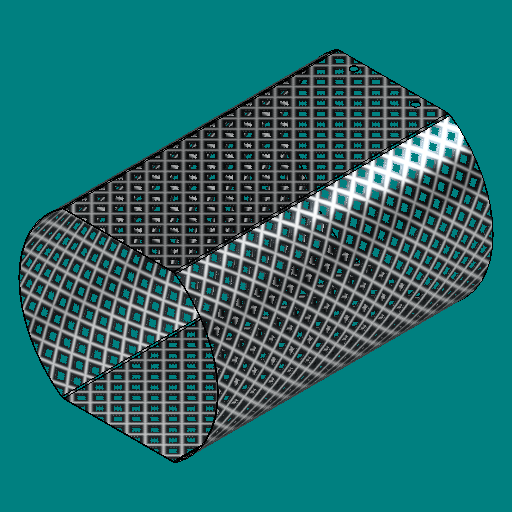
# Autodesk Inventor part: probe-side-large-mesh
Saved by Autodesk Inventor 2025 (Build 290162000, 162)
## iProperties
Created: 2024-05-22
Part Number: probe-side-large-mesh
Material: Stainless Steel
Document SubType Name: Modeling
Designer: kuzmin
Density: 8 g/cm^3
Appearance: Expanded Metal 02
Author: kuzmin
Autodesk Inventor part; units mm, degrees
ref_plane "YZ Plane" through (0, 0, 0) normal (1, 0, 0) x (0, 1, 0)
ref_plane "XZ Plane" through (0, 0, 0) normal (0, 1, 0) x (-1, 0, 0)
ref_plane "XY Plane" through (0, 0, 0) normal (0, 0, 1) x (1, 0, 0)
sketch "Sketch1" plane through (0, 0, 0) normal (0, 0, 1) x (1, 0, 0)
  circle A0 centre (0, 0) radius 28.8
  line L0 (-50, 23.8) -> (50, 23.8)
  line L1 (50, 23.8) -> (50, -23.8)
  line L2 (50, -23.8) -> (-50, -23.8)
  line L3 (-50, -23.8) -> (-50, 23.8)
  point P0 (50, 0)
  point P1 (0, 23.8)
  point P2 (-16.217275, -23.8)
  point P3 (16.217275, -23.8)
  point P4 (16.217275, 23.8)
  point P5 (-16.217275, 23.8)
  dimension "d0" = 57.6
  dimension "d1" = 47.6
  dimension "d2" = 100
  constraints: 8 end point, 2 midpoint, 2 parallel, 1 centre point, 1 coincident, 1 horizontal, 1 horizontal alignment, 1 perpendicular, 1 vertical alignment
  measures "d0" diameter of A0
  measures "d1" distance between parallel lines of L2 L0
  measures "d2" distance of L0.start L0.end
sketch "Sketch1 outline for Extrusion1" plane through (0, 0, 0) normal (0, 0, 1) x (1, 0, 0)
  line L0 (-16.217275, -23.8) -> (16.217275, -23.8)
  arc A0 (-16.217275, 23.8) -> (-16.217275, -23.8) centre (0, 0) ccw
  line L1 (16.217275, 23.8) -> (-16.217275, 23.8)
  arc A1 (16.217275, -23.8) -> (16.217275, 23.8) centre (0, 0) ccw
extrude "Extrusion1" add sketch "Sketch1 outline for Extrusion1" along normal blind 80
fillet "Fillet1" radius 1 4 edges at (-16.2173, 23.8, 40) (16.2173, 23.8, 40) (16.2173, -23.8, 40) (-16.2173, -23.8, 40)
thicken "Thicken1" operation add thickness 0.2 both sides no extend neighbours no toward (0, 1, 0) faces at (5.301991, 23.8, 26.666667) (-16.040924, 23.790852, 26.666667) (-27.332956, -9.074665, 53.333333) (16.237959, 23.743284, 26.666667) (28.430873, 4.596242, 53.333333) (16.362219, -23.689854, 26.666667) (-5.301991, -23.8, 26.666667) (-16.362219, -23.689854, 26.666667)
shell "Shell1" thickness 0.2 removed faces 2 at (-5.301991, -8, 80) at (-5.301991, -8, 0)
sketch "Sketch2" plane through (-19.580613, 24, 0) normal (0, 1, 0) x (1, 0, 0)
  line L0 (10.580613, -2.5) -> (28.580613, -2.5) construction
  line L1 (35.486587, 0) -> (3.674639, 0)
  point P0 (19.580613, 0)
  point P1 (31.432467, 0)
  point P2 (0, 0)
  point P3 (19.580613, -2.5)
  point P4 (19.580613, 0)
  point P5 (27.757828, 0)
  point P6 (19.580613, 0)
  dimension "d9" = 18
  dimension "d10" = 2.5
  constraints: 3 midpoint, 2 coincident, 2 end point, 2 vertical alignment, 1 horizontal
  measures "d9" distance of L0.start L0.end
  measures "d10" distance between parallel lines of L1 L0
hole "Hole1" at (-9, 24, 2.5) at (9, 24, 2.5) direction (0, -1, 0) diameter 2.1 end through all
equation "\"d0\" = phi + 2 * slack"
equation "\"d1\" = flat_width + 2 * slack"
equation "\"flat_width\" = 44"
equation "\"phi\" = 54"
equation "\"slack\" = 1.8"
body "Solid1"
